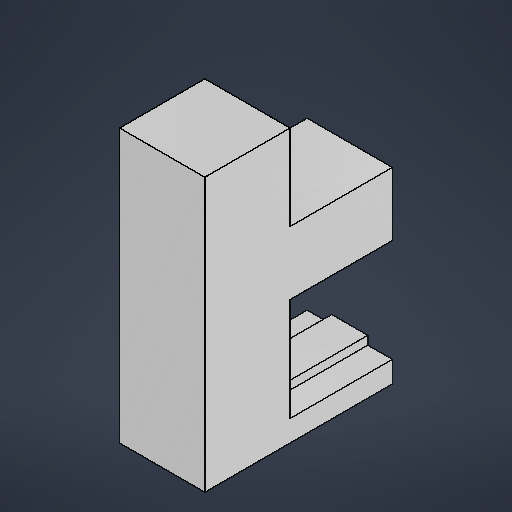
# Autodesk Inventor part: A Idler
Saved by Autodesk Inventor 2026 (Build 300175050, 175E)
## iProperties
Created: 2025-04-15
Part Number: A Idler
Material: Aluminum 6061
Document SubType Name: Modeling
Designer: Joshua Eah
Density: 2.7 g/cm^3
Appearance: Machined - Aluminum
Author: Joshua Eah
Autodesk Inventor part; units mm, degrees
ref_plane "YZ Plane" through (0, 0, 0) normal (1, 0, 0) x (0, 1, 0)
ref_plane "XZ Plane" through (0, 0, 0) normal (0, 1, 0) x (-1, 0, 0)
ref_plane "XY Plane" through (0, 0, 0) normal (0, 0, 1) x (1, 0, 0)
sketch "Base Profile" plane through (0, 0, 0) normal (0, 1, 0) x (-1, 0, 0)
  line L0 (0, 0) -> (15, 0)
  line L1 (15, 0) -> (15, -15)
  line L2 (15, -15) -> (0, -15)
  line L3 (0, -15) -> (0, 0)
  line L4 (15, 0) -> (33, 0)
  line L5 (33, 0) -> (33, -15)
  line L6 (33, -15) -> (15, -15)
  line L7 (15, -15) -> (15, 0)
  dimension "d164" = 15
  dimension "d165" = 15
  dimension "d166" = 18
  dimension "d167" = 15
  constraints: 16 end point, 4 parallel, 2 horizontal, 2 perpendicular, 2 point on line
  measures "d164" distance of L1.end L2.end
  measures "d165" distance of L0.end L1.end
  measures "d166" distance of L5.end L6.end
  measures "d167" distance of L4.end L5.end
extrude "Stock" add sketch "Base Profile" against normal blind 33
extrude "Extrusion Post" add sketch "Base Profile" along normal blind 15 contours L0 L1 L2 L3
sketch "Slot Cutout" plane through (-33, 0, -15) normal (-1, 0, 0) x (0, 0, 1)
  line L0 (0, 0) -> (15, 0) construction
  line L1 (7.5, 0) -> (7.5, -33) construction
  line L2 (15, -33) -> (0, -33) construction
  line L3 (0, 0) -> (0, -33) projected
  line L4 (15, 0) -> (15, -33) projected
  line L5 (0, -29.25) -> (15, -29.25)
  line L6 (0, -11.1439) -> (15, -11.1439)
  line L7 (4.325, -27.75) -> (10.675, -27.75)
  line L8 (10.675, -27.75) -> (10.675, -29.25)
  line L9 (10.675, -29.25) -> (4.325, -29.25)
  line L10 (4.325, -29.25) -> (4.325, -27.75)
  line L11 (4.325, -27.75) -> (10.675, -29.25) construction
  line L12 (10.675, -27.75) -> (4.325, -29.25) construction
  point P0 (7.5, -28.5)
  dimension "d355" = 3.75
  dimension "d356" = 6.35
  dimension "d357" = 1.5
  dimension "d317" = 6.35
  dimension "d318" = 7.5
  dimension "d319" = 7.5
  constraints: 18 end point, 6 point on line, 4 midpoint, 3 perpendicular, 2 parallel, 1 horizontal
  measures "d355" distance between parallel lines of L2 L5
  measures "d356" distance of L8.end L9.end
  measures "d357" distance of L9.end L7.start
extrude "Extrusion18" cut sketch "Slot Cutout" against normal up to surface (18 mm away) contours L6 L4 L5 L8 L7 L10 L3
equation "\"d164\" = extrusionWidth"
equation "\"d165\" = extrusionWidth"
equation "\"d166\" = idlerLength"
equation "\"d167\" = d165"
equation "\"d168\" = extrusionOffset"
equation "\"extrusionWidth\" = 15"
equation "\"idlerLength\" = 18"
equation "\"bearingOffsetFromBottom\" = 7.5"
equation "\"extrusionOffset\" = 33"
equation "\"bearingStackHeight\" = 9"
equation "\"bearingSlotLength\" = 5"
equation "\"bearingClearance\" = 13"
equation "\"pinSupportLength\" = 2"
body "Solid2"
